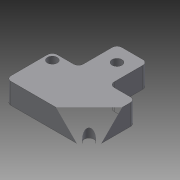
# Autodesk Inventor part: EndStop_Bracket
Saved by Autodesk Inventor 2014 (Build 180170000, 170)
## iProperties
Created: 2014-03-22
Part Number: EndStop_Bracket
Material: Generic
Document SubType Name: Modeling
Designer: ThatOtherGuy
Density: 1 g/cm^3
Appearance: Default
Author: ThatOtherGuy
Autodesk Inventor part; units mm, degrees
ref_plane "YZ Plane" through (0, 0, 0) normal (1, 0, 0) x (0, 1, 0)
ref_plane "XZ Plane" through (0, 0, 0) normal (0, 1, 0) x (-1, 0, 0)
ref_plane "XY Plane" through (0, 0, 0) normal (0, 0, 1) x (1, 0, 0)
sketch "Sketch1" plane through (0, 0, 0) normal (0, 0, 1) x (1, 0, 0)
  circle A0 centre (13.45, 22.5) radius 1.59
  circle A1 centre (2.35, 12.65) radius 1.59
  circle A2 centre (24.55, 2.35) radius 1.59
  line L0 (0, 0) -> (0, 15)
  line L1 (0, 15) -> (8.45, 15)
  line L2 (8.45, 15) -> (8.45, 27.5)
  line L3 (8.45, 27.5) -> (18.45, 27.5)
  line L4 (18.45, 27.5) -> (18.45, 15)
  line L5 (18.45, 15) -> (26.9, 15)
  line L6 (26.9, 15) -> (26.9, 0)
  line L7 (26.9, 0) -> (0, 0)
  point P0 (13.45, 27.5)
  dimension "d8" = 3.18
  dimension "d9" = 10.3
  dimension "d10" = 22.2
  dimension "d18" = 15
  dimension "d19" = 2.35
  dimension "d20" = 2.35
  dimension "d21" = 2.35
  dimension "d22" = 2.35
  dimension "d24" = 26.9
  dimension "d27" = 5
  dimension "d30" = 12.5
  dimension "d32" = 10
  dimension "d33" = 8.45
  dimension "d34" = 8.45
  constraints: 16 end point, 6 parallel, 3 centre point, 2 equal radius, 1 collinear, 1 midpoint, 1 perpendicular, 1 vertical, 1 vertical alignment
  measures "d8" diameter of A2
  measures "d9" vertical distance of A1.centre A2.centre
  measures "d10" horizontal distance of A1.centre A2.centre
  measures "d18" distance of L5.end L6.end
  measures "d19" distance from line of L7 A2.centre
  measures "d20" distance from line of L6 A2.centre
  measures "d21" distance from line of L0 A1.centre
  measures "d22" distance from line of L1 A1.centre
  measures "d24" distance between parallel lines of L0 L6
  measures "d27" distance from line of L3 A0.centre
  measures "d30" distance of L1.end L2.end
  measures "d32" distance of L2.end L3.end
  measures "d33" distance between parallel lines of L0 L2
  measures "d34" distance of L4.end L5.end
extrude "Extrusion1" add sketch "Sketch1" along normal blind 6.731
fillet "Fillet1" radius 1.5875 8 edges at (18.45, 15, 3.3655) (8.45, 15, 3.3655) (0, 0, 3.3655) (26.9, 0, 3.3655) (0, 15, 3.3655) (8.45, 27.5, 3.3655) (18.45, 27.5, 3.3655) (26.9, 15, 3.3655)
equation "\"d19\" = d22"
equation "\"d20\" = d19"
equation "\"d21\" = d19"
equation "\"d33\" = d34"
equation "\"d2\" = THICKB"
equation "\"THICKA\" = 3.175"
equation "\"THICKB\" = 6.731"
equation "\"THICKC\" = 12.7"
equation "\"BALLDIA\" = 12"
equation "\"MAGDIA\" = 9.5"
equation "\"THICKPLY\" = 5"
body "Solid1"
